Autodesk Inventor part; units mm, degrees
(part 2 of 3)
  spline S198 degree 2 poles (343.738, 65.1284) (343.9064, 65.1284) (344.2478, 65.1557) (344.571, 65.2012) (344.8623, 65.2604) (344.9852, 65.2968) knots 0 0 0 1 2 3 4 4 4
  line L272 (344.9852, 65.2968) -> (344.9852, 64.7415)
  spline S199 degree 2 poles (344.9852, 64.7415) (344.7076, 64.6641) (344.0111, 64.564) (343.6379, 64.564) knots 0 0 0 1 2 2 2
  spline S200 degree 2 poles (343.6379, 64.564) (343.1371, 64.564) (342.4134, 64.8371) (341.9536, 65.3515) (341.7306, 66.1025) (341.7306, 66.5759) knots 0 0 0 1 2 3 4 4 4
  spline S201 degree 2 poles (341.7306, 66.5759) (341.7306, 66.9902) (341.9673, 67.723) (342.4225, 68.2784) (343.0825, 68.6061) (343.5013, 68.6061) knots 0 0 0 1 2 3 4 4 4
  spline S202 degree 2 poles (343.5013, 68.6061) (343.911, 68.6061) (344.5437, 68.3512) (344.9716, 67.8778) (345.1946, 67.2087) (345.1946, 66.7899) knots 0 0 0 1 2 3 4 4 4
  spline S203 degree 2 poles (344.4891, 66.8855) (344.5027, 67.1449) (344.3753, 67.5774) (344.1158, 67.8915) (343.7289, 68.0644) (343.4694, 68.0644) knots 0 0 0 1 2 3 4 4 4
  spline S204 degree 2 poles (343.4694, 68.0644) (343.2509, 68.0644) (342.8822, 67.8915) (342.6182, 67.5819) (342.4543, 67.1449) (342.4361, 66.8855) knots 0 0 0 1 2 3 4 4 4
  line L273 (342.4361, 66.8855) -> (344.4891, 66.8855)
  spline S205 degree 2 poles (346.0777, 66.5031) (346.0777, 66.9993) (346.3508, 67.7731) (346.8515, 68.3057) (347.5525, 68.5834) (347.985, 68.5834) knots 0 0 0 1 2 3 4 4 4
  spline S206 degree 2 poles (347.985, 68.5834) (348.1716, 68.5834) (348.5358, 68.5378) (348.7087, 68.4878) knots 0 0 0 1 2 2 2
  line L274 (348.7087, 68.4878) -> (348.7087, 70.1265)
  line L275 (348.7087, 70.1265) -> (349.387, 70.1265)
  line L276 (349.387, 70.1265) -> (349.387, 64.6322)
  line L277 (349.387, 64.6322) -> (348.7816, 64.6322)
  line L278 (348.7816, 64.6322) -> (348.7588, 65.3742)
  spline S207 degree 2 poles (348.7588, 65.3742) (348.4766, 64.96) (347.8166, 64.564) (347.4296, 64.564) knots 0 0 0 1 2 2 2
  spline S208 degree 2 poles (347.4296, 64.564) (347.0973, 64.564) (346.5875, 64.8416) (346.2507, 65.3515) (346.0777, 66.0661) (346.0777, 66.5031) knots 0 0 0 1 2 3 4 4 4
  spline S209 degree 2 poles (346.7696, 66.5441) (346.7696, 65.8385) (347.1838, 65.1421) (347.5662, 65.1421) knots 0 0 0 1 2 2 2
  spline S210 degree 2 poles (347.5662, 65.1421) (347.8211, 65.1421) (348.3947, 65.6018) (348.7087, 66.0525) knots 0 0 0 1 2 2 2
  line L279 (348.7087, 66.0525) -> (348.7087, 67.8641)
  spline S211 degree 2 poles (348.7087, 67.8641) (348.5403, 67.9415) (348.1398, 68.0235) (347.9395, 68.0235) knots 0 0 0 1 2 2 2
  spline S212 degree 2 poles (347.9395, 68.0235) (347.3887, 68.0235) (346.7696, 67.3088) (346.7696, 66.5441) knots 0 0 0 1 2 2 2
  spline S213 degree 2 poles (358.3726, 66.6533) (358.3726, 66.1708) (358.104, 65.4015) (357.6124, 64.8689) (356.9023, 64.5867) (356.4608, 64.5867) knots 0 0 0 1 2 3 4 4 4
  spline S214 degree 2 poles (356.4608, 64.5867) (356.1148, 64.5867) (355.391, 64.7187) (355.036, 64.8644) knots 0 0 0 1 2 2 2
  line L280 (355.036, 64.8644) -> (355.036, 70.1265)
  line L281 (355.036, 70.1265) -> (355.7142, 70.1265)
  line L282 (355.7142, 70.1265) -> (355.7142, 68.6152)
  line L283 (355.7142, 68.6152) -> (355.6824, 67.8915)
  spline S215 degree 2 poles (355.6824, 67.8915) (355.9737, 68.2829) (356.6383, 68.6061) (357.0206, 68.6061) knots 0 0 0 1 2 2 2
  spline S216 degree 2 poles (357.0206, 68.6061) (357.3529, 68.6061) (357.8582, 68.3284) (358.1996, 67.8186) (358.3726, 67.0994) (358.3726, 66.6533) knots 0 0 0 1 2 3 4 4 4
  spline S217 degree 2 poles (357.6807, 66.6215) (357.6807, 66.931) (357.5896, 67.4408) (357.3985, 67.8095) (357.0935, 68.0144) (356.8841, 68.0144) knots 0 0 0 1 2 3 4 4 4
  spline S218 degree 2 poles (356.8841, 68.0144) (356.7566, 68.0144) (356.4926, 67.9324) (356.2058, 67.7412) (355.8918, 67.4272) (355.7142, 67.195) knots 0 0 0 1 2 3 4 4 4
  line L284 (355.7142, 67.195) -> (355.7142, 65.3014)
  spline S219 degree 2 poles (355.7142, 65.3014) (355.9145, 65.224) (356.3242, 65.133) (356.5108, 65.133) knots 0 0 0 1 2 2 2
  spline S220 degree 2 poles (356.5108, 65.133) (356.743, 65.133) (357.1663, 65.2786) (357.4895, 65.6246) (357.6807, 66.1981) (357.6807, 66.6215) knots 0 0 0 1 2 3 4 4 4
  line L285 (362.8881, 68.5333) -> (361.559, 65.0465)
  spline S221 degree 2 poles (361.559, 65.0465) (361.3496, 64.5139) (360.9126, 63.7446) (360.3891, 63.2484) (359.77, 63.0163) (359.3831, 63.0163) knots 0 0 0 1 2 3 4 4 4
  spline S222 degree 2 poles (359.3831, 63.0163) (359.283, 63.0163) (359.1191, 63.0254) (359.0235, 63.0345) knots 0 0 0 1 2 2 2
  line L286 (359.0235, 63.0345) -> (359.0235, 63.649)
  spline S223 degree 2 poles (359.0235, 63.649) (359.1055, 63.6354) (359.3103, 63.6172) (359.4241, 63.6172) knots 0 0 0 1 2 2 2
  spline S224 degree 2 poles (359.4241, 63.6172) (359.6107, 63.6172) (359.9339, 63.7264) (360.2207, 63.9677) (360.4847, 64.3591) (360.6076, 64.6322) knots 0 0 0 1 2 3 4 4 4
  line L287 (360.6076, 64.6322) -> (359.0508, 68.5333)
  line L288 (359.0508, 68.5333) -> (359.8201, 68.5333)
  line L289 (359.8201, 68.5333) -> (360.8079, 65.9523)
  line L290 (360.8079, 65.9523) -> (361.0082, 65.3469)
  line L291 (361.0082, 65.3469) -> (361.2312, 65.9705)
  line L292 (361.2312, 65.9705) -> (362.1416, 68.5333)
  line L293 (362.1416, 68.5333) -> (362.8881, 68.5333)
  line L294 (371.7508, 69.7122) -> (371.4094, 64.6322)
  line L295 (371.4094, 64.6322) -> (370.5127, 64.6322)
  line L296 (370.5127, 64.6322) -> (369.88, 66.4394)
  line L297 (369.88, 66.4394) -> (369.707, 67.0175)
  line L298 (369.707, 67.0175) -> (369.5249, 66.3939)
  line L299 (369.5249, 66.3939) -> (368.9377, 64.6322)
  line L300 (368.9377, 64.6322) -> (368.0728, 64.6322)
  line L301 (368.0728, 64.6322) -> (367.7223, 69.7122)
  line L302 (367.7223, 69.7122) -> (368.3733, 69.7122)
  line L303 (368.3733, 69.7122) -> (368.5736, 66.2527)
  line L304 (368.5736, 66.2527) -> (368.6327, 65.3059)
  line L305 (368.6327, 65.3059) -> (368.8785, 66.1116)
  line L306 (368.8785, 66.1116) -> (369.493, 67.9962)
  line L307 (369.493, 67.9962) -> (369.971, 67.9962)
  line L308 (369.971, 67.9962) -> (370.6811, 65.9751)
  line L309 (370.6811, 65.9751) -> (370.9178, 65.3059)
  line L310 (370.9178, 65.3059) -> (370.9315, 66.0024)
  line L311 (370.9315, 66.0024) -> (371.1318, 69.7122)
  line L312 (371.1318, 69.7122) -> (371.7508, 69.7122)
  line L313 (373.8811, 67.9734) -> (372.7249, 67.9734)
  line L314 (372.7249, 67.9734) -> (372.7249, 68.5333)
  line L315 (372.7249, 68.5333) -> (374.5639, 68.5333)
  line L316 (374.5639, 68.5333) -> (374.5639, 65.1967)
  line L317 (374.5639, 65.1967) -> (375.7247, 65.1967)
  line L318 (375.7247, 65.1967) -> (375.7247, 64.6322)
  line L319 (375.7247, 64.6322) -> (372.5975, 64.6322)
  line L320 (372.5975, 64.6322) -> (372.5975, 65.1967)
  line L321 (372.5975, 65.1967) -> (373.8811, 65.1967)
  line L322 (373.8811, 65.1967) -> (373.8811, 67.9734)
  spline S225 degree 2 poles (374.1179, 70.172) (374.2317, 70.172) (374.4228, 70.0901) (374.5685, 69.9444) (374.6504, 69.7532) (374.6504, 69.6394) knots 0 0 0 1 2 3 4 4 4
  spline S226 degree 2 poles (374.6504, 69.6394) (374.6504, 69.5302) (374.5685, 69.3344) (374.4228, 69.1888) (374.2317, 69.1068) (374.1179, 69.1068) knots 0 0 0 1 2 3 4 4 4
  spline S227 degree 2 poles (374.1179, 69.1068) (374.0041, 69.1068) (373.8129, 69.1888) (373.6672, 69.3344) (373.5853, 69.5302) (373.5853, 69.6394) knots 0 0 0 1 2 3 4 4 4
  spline S228 degree 2 poles (373.5853, 69.6394) (373.5853, 69.7532) (373.6672, 69.9444) (373.8129, 70.0901) (374.0041, 70.172) (374.1179, 70.172) knots 0 0 0 1 2 3 4 4 4
  line L323 (376.931, 68.5333) -> (377.5364, 68.5333)
  line L324 (377.5364, 68.5333) -> (377.5637, 67.9051)
  spline S229 degree 2 poles (377.5637, 67.9051) (377.7321, 68.1054) (378.0508, 68.374) (378.3603, 68.5378) (378.6789, 68.6061) (378.8519, 68.6061) knots 0 0 0 1 2 3 4 4 4
  spline S230 degree 2 poles (378.8519, 68.6061) (379.4528, 68.6061) (380.0718, 67.896) (380.0718, 67.1813) knots 0 0 0 1 2 2 2
  line L325 (380.0718, 67.1813) -> (380.0718, 64.6322)
  line L326 (380.0718, 64.6322) -> (379.3936, 64.6322)
  line L327 (379.3936, 64.6322) -> (379.3936, 67.1267)
  spline S231 degree 2 poles (379.3936, 67.1267) (379.3936, 67.5819) (379.0522, 68.0235) (378.7153, 68.0235) knots 0 0 0 1 2 2 2
  spline S232 degree 2 poles (378.7153, 68.0235) (378.5879, 68.0235) (378.3512, 67.9506) (378.0963, 67.7686) (377.7958, 67.4545) (377.6092, 67.2223) knots 0 0 0 1 2 3 4 4 4
  line L328 (377.6092, 67.2223) -> (377.6092, 64.6322)
  line L329 (377.6092, 64.6322) -> (376.931, 64.6322)
  line L330 (376.931, 64.6322) -> (376.931, 68.5333)
  spline S233 degree 2 poles (381.1097, 66.5031) (381.1097, 66.9993) (381.3828, 67.7731) (381.8835, 68.3057) (382.5845, 68.5834) (383.017, 68.5834) knots 0 0 0 1 2 3 4 4 4
  spline S234 degree 2 poles (383.017, 68.5834) (383.2036, 68.5834) (383.5677, 68.5378) (383.7407, 68.4878) knots 0 0 0 1 2 2 2
  line L331 (383.7407, 68.4878) -> (383.7407, 70.1265)
  line L332 (383.7407, 70.1265) -> (384.419, 70.1265)
  line L333 (384.419, 70.1265) -> (384.419, 64.6322)
  line L334 (384.419, 64.6322) -> (383.8136, 64.6322)
  line L335 (383.8136, 64.6322) -> (383.7908, 65.3742)
  spline S235 degree 2 poles (383.7908, 65.3742) (383.5086, 64.96) (382.8485, 64.564) (382.4616, 64.564) knots 0 0 0 1 2 2 2
  spline S236 degree 2 poles (382.4616, 64.564) (382.1293, 64.564) (381.6195, 64.8416) (381.2827, 65.3515) (381.1097, 66.0661) (381.1097, 66.5031) knots 0 0 0 1 2 3 4 4 4
  spline S237 degree 2 poles (381.8016, 66.5441) (381.8016, 65.8385) (382.2158, 65.1421) (382.5982, 65.1421) knots 0 0 0 1 2 2 2
  spline S238 degree 2 poles (382.5982, 65.1421) (382.8531, 65.1421) (383.4266, 65.6018) (383.7407, 66.0525) knots 0 0 0 1 2 2 2
  line L336 (383.7407, 66.0525) -> (383.7407, 67.8641)
  spline S239 degree 2 poles (383.7407, 67.8641) (383.5723, 67.9415) (383.1717, 68.0235) (382.9714, 68.0235) knots 0 0 0 1 2 2 2
  spline S240 degree 2 poles (382.9714, 68.0235) (382.4206, 68.0235) (381.8016, 67.3088) (381.8016, 66.5441) knots 0 0 0 1 2 2 2
  spline S241 degree 2 poles (389.2304, 67.2087) (389.2304, 66.5213) (388.9072, 65.529) (388.361, 64.8781) (387.6236, 64.564) (387.2184, 64.564) knots 0 0 0 1 2 3 4 4 4
  spline S242 degree 2 poles (387.2184, 64.564) (386.7268, 64.564) (385.9985, 64.919) (385.5205, 65.5882) (385.2884, 66.5486) (385.2884, 67.1495) knots 0 0 0 1 2 3 4 4 4
  spline S243 degree 2 poles (385.2884, 67.1495) (385.2884, 67.8277) (385.607, 68.8201) (386.1533, 69.471) (386.8861, 69.7851) (387.2958, 69.7851) knots 0 0 0 1 2 3 4 4 4
  spline S244 degree 2 poles (387.2958, 69.7851) (387.7829, 69.7851) (388.5112, 69.4255) (388.9937, 68.7609) (389.2304, 67.805) (389.2304, 67.2087) knots 0 0 0 1 2 3 4 4 4
  spline S245 degree 2 poles (388.5385, 67.1586) (388.5385, 67.6047) (388.3974, 68.3467) (388.0879, 68.8838) (387.6008, 69.1797) (387.2548, 69.1797) knots 0 0 0 1 2 3 4 4 4
  spline S246 degree 2 poles (387.2548, 69.1797) (386.9225, 69.1797) (386.44, 68.8656) (386.1305, 68.3239) (385.9803, 67.5956) (385.9803, 67.1859) knots 0 0 0 1 2 3 4 4 4
  spline S247 degree 2 poles (385.9803, 67.1859) (385.9803, 66.7353) (386.1214, 65.9933) (386.4309, 65.4607) (386.9134, 65.1648) (387.2548, 65.1648) knots 0 0 0 1 2 3 4 4 4
  spline S248 degree 2 poles (387.2548, 65.1648) (387.5871, 65.1648) (388.0742, 65.4789) (388.3883, 66.0206) (388.5385, 66.7444) (388.5385, 67.1586) knots 0 0 0 1 2 3 4 4 4
  spline S249 degree 2 poles (393.3181, 66.0115) (393.3181, 65.6473) (393.0222, 65.1056) (392.4942, 64.7415) (391.7522, 64.564) (391.3015, 64.564) knots 0 0 0 1 2 3 4 4 4
  spline S250 degree 2 poles (391.3015, 64.564) (391.1013, 64.564) (390.7007, 64.5958) (390.332, 64.6413) (390.0042, 64.7005) (389.8722, 64.7369) knots 0 0 0 1 2 3 4 4 4
  line L337 (389.8722, 64.7369) -> (389.8722, 65.4061)
  spline S251 degree 2 poles (389.8722, 65.4061) (390.1636, 65.2968) (390.8919, 65.1739) (391.3516, 65.1739) knots 0 0 0 1 2 2 2
  spline S252 degree 2 poles (391.3516, 65.1739) (391.6885, 65.1739) (392.1573, 65.2786) (392.4577, 65.4835) (392.5943, 65.7793) (392.5943, 65.9705) knots 0 0 0 1 2 3 4 4 4
  spline S253 degree 2 poles (392.5943, 65.9705) (392.5943, 66.1754) (392.3667, 66.4667) (391.9934, 66.6988) (391.5155, 66.89) (391.0148, 67.0903) (390.5368, 67.327) (390.1636, 67.6502) (389.936, 68.0872) (389.936, 68.3876) knots 0 0 0 1 2 3 4 5 6 7 8 8 8
  spline S254 degree 2 poles (389.936, 68.3876) (389.936, 68.6471) (390.1544, 69.1524) (390.6142, 69.5438) (391.3289, 69.7851) (391.8296, 69.7851) knots 0 0 0 1 2 3 4 4 4
  spline S255 degree 2 poles (391.8296, 69.7851) (391.957, 69.7851) (392.2575, 69.7623) (392.5624, 69.7213) (392.8629, 69.6667) (392.9903, 69.6349) knots 0 0 0 1 2 3 4 4 4
  line L338 (392.9903, 69.6349) -> (392.9903, 69.0112)
  spline S256 degree 2 poles (392.9903, 69.0112) (392.6899, 69.0977) (392.0936, 69.1842) (391.8114, 69.1842) knots 0 0 0 1 2 2 2
  spline S257 degree 2 poles (391.8114, 69.1842) (391.2196, 69.1842) (390.6597, 68.7882) (390.6597, 68.4559) knots 0 0 0 1 2 2 2
  spline S258 degree 2 poles (390.6597, 68.4559) (390.6597, 68.2511) (390.8873, 67.9552) (391.2606, 67.7185) (391.7385, 67.5319) (392.2393, 67.327) (392.7172, 67.0858) (393.0905, 66.758) (393.3181, 66.3119) (393.3181, 66.0115) knots 0 0 0 1 2 3 4 5 6 7 8 8 8
  line L339 (323.723, 56.0664) -> (322.9673, 56.0664)
  line L340 (322.9673, 56.0664) -> (322.6168, 57.1726)
  line L341 (322.6168, 57.1726) -> (320.4911, 57.1726)
  line L342 (320.4911, 57.1726) -> (320.136, 56.0664)
  line L343 (320.136, 56.0664) -> (319.4214, 56.0664)
  line L344 (319.4214, 56.0664) -> (321.1056, 61.1464)
  line L345 (321.1056, 61.1464) -> (322.057, 61.1464)
  line L346 (322.057, 61.1464) -> (323.723, 56.0664)
  line L347 (322.4166, 57.7916) -> (321.5562, 60.5137)
  line L348 (321.5562, 60.5137) -> (320.6868, 57.7916)
  line L349 (320.6868, 57.7916) -> (322.4166, 57.7916)
  spline S259 degree 2 poles (327.4692, 57.1316) (327.4692, 56.9268) (327.3281, 56.599) (327.0869, 56.3487) (326.7682, 56.1711) (326.4086, 56.0528) (326.0263, 55.9982) (325.8442, 55.9982) knots 0 0 0 1 2 3 4 5 6 6 6
  spline S260 degree 2 poles (325.8442, 55.9982) (325.4482, 55.9982) (324.7836, 56.071) (324.4649, 56.1484) knots 0 0 0 1 2 2 2
  line L350 (324.4649, 56.1484) -> (324.4649, 56.772)
  spline S261 degree 2 poles (324.4649, 56.772) (324.8063, 56.6718) (325.4846, 56.5717) (325.8169, 56.5717) knots 0 0 0 1 2 2 2
  spline S262 degree 2 poles (325.8169, 56.5717) (326.3039, 56.5717) (326.7682, 56.8357) (326.7682, 57.077) knots 0 0 0 1 2 2 2
  spline S263 degree 2 poles (326.7682, 57.077) (326.7682, 57.1817) (326.6954, 57.3501) (326.4997, 57.5003) (326.0946, 57.6642) (325.7395, 57.7689) knots 0 0 0 1 2 3 4 4 4
  spline S264 degree 2 poles (325.7395, 57.7689) (325.4755, 57.8463) (325.0294, 58.0465) (324.7016, 58.3197) (324.515, 58.6838) (324.515, 58.9342) knots 0 0 0 1 2 3 4 4 4
  spline S265 degree 2 poles (324.515, 58.9342) (324.515, 59.098) (324.6652, 59.485) (325.0339, 59.8173) (325.653, 60.0403) (326.1219, 60.0403) knots 0 0 0 1 2 3 4 4 4
  spline S266 degree 2 poles (326.1219, 60.0403) (326.3495, 60.0403) (326.9094, 59.9902) (327.2143, 59.9265) knots 0 0 0 1 2 2 2
  line L351 (327.2143, 59.9265) -> (327.2143, 59.3256)
  spline S267 degree 2 poles (327.2143, 59.3256) (326.8957, 59.403) (326.3222, 59.4759) (326.1128, 59.4759) knots 0 0 0 1 2 2 2
  spline S268 degree 2 poles (326.1128, 59.4759) (325.8624, 59.4759) (325.5165, 59.3985) (325.3025, 59.2619) (325.2069, 59.0798) (325.2069, 58.9751) knots 0 0 0 1 2 3 4 4 4
  spline S269 degree 2 poles (325.2069, 58.9751) (325.2069, 58.8704) (325.2889, 58.6975) (325.5119, 58.5382) (325.9079, 58.3788) (326.2266, 58.2878) knots 0 0 0 1 2 3 4 4 4
  spline S270 degree 2 poles (326.2266, 58.2878) (326.5725, 58.1877) (327.0459, 57.9646) (327.3418, 57.6915) (327.4692, 57.3501) (327.4692, 57.1316) knots 0 0 0 1 2 3 4 4 4
  spline S271 degree 2 poles (331.8482, 57.1316) (331.8482, 56.9268) (331.7071, 56.599) (331.4659, 56.3487) (331.1472, 56.1711) (330.7876, 56.0528) (330.4053, 55.9982) (330.2232, 55.9982) knots 0 0 0 1 2 3 4 5 6 6 6
  spline S272 degree 2 poles (330.2232, 55.9982) (329.8272, 55.9982) (329.1626, 56.071) (328.8439, 56.1484) knots 0 0 0 1 2 2 2
  line L352 (328.8439, 56.1484) -> (328.8439, 56.772)
  spline S273 degree 2 poles (328.8439, 56.772) (329.1853, 56.6718) (329.8636, 56.5717) (330.1959, 56.5717) knots 0 0 0 1 2 2 2
  spline S274 degree 2 poles (330.1959, 56.5717) (330.6829, 56.5717) (331.1472, 56.8357) (331.1472, 57.077) knots 0 0 0 1 2 2 2
  spline S275 degree 2 poles (331.1472, 57.077) (331.1472, 57.1817) (331.0744, 57.3501) (330.8787, 57.5003) (330.4735, 57.6642) (330.1185, 57.7689) knots 0 0 0 1 2 3 4 4 4
  spline S276 degree 2 poles (330.1185, 57.7689) (329.8545, 57.8463) (329.4084, 58.0465) (329.0806, 58.3197) (328.894, 58.6838) (328.894, 58.9342) knots 0 0 0 1 2 3 4 4 4
  spline S277 degree 2 poles (328.894, 58.9342) (328.894, 59.098) (329.0442, 59.485) (329.4129, 59.8173) (330.032, 60.0403) (330.5009, 60.0403) knots 0 0 0 1 2 3 4 4 4
  spline S278 degree 2 poles (330.5009, 60.0403) (330.7285, 60.0403) (331.2884, 59.9902) (331.5933, 59.9265) knots 0 0 0 1 2 2 2
  line L353 (331.5933, 59.9265) -> (331.5933, 59.3256)
  spline S279 degree 2 poles (331.5933, 59.3256) (331.2747, 59.403) (330.7011, 59.4759) (330.4918, 59.4759) knots 0 0 0 1 2 2 2
  spline S280 degree 2 poles (330.4918, 59.4759) (330.2414, 59.4759) (329.8954, 59.3985) (329.6815, 59.2619) (329.5859, 59.0798) (329.5859, 58.9751) knots 0 0 0 1 2 3 4 4 4
  spline S281 degree 2 poles (329.5859, 58.9751) (329.5859, 58.8704) (329.6679, 58.6975) (329.8909, 58.5382) (330.2869, 58.3788) (330.6056, 58.2878) knots 0 0 0 1 2 3 4 4 4
  spline S282 degree 2 poles (330.6056, 58.2878) (330.9515, 58.1877) (331.4249, 57.9646) (331.7208, 57.6915) (331.8482, 57.3501) (331.8482, 57.1316) knots 0 0 0 1 2 3 4 4 4
  spline S283 degree 2 poles (336.4366, 58.2241) (336.4366, 58.083) (336.4275, 57.8872) (336.423, 57.8007) knots 0 0 0 1 2 2 2
  line L354 (336.423, 57.8007) -> (333.6781, 57.8007)
  spline S284 degree 2 poles (333.6781, 57.8007) (333.6781, 57.2044) (334.3473, 56.5626) (334.98, 56.5626) knots 0 0 0 1 2 2 2
  spline S285 degree 2 poles (334.98, 56.5626) (335.1484, 56.5626) (335.4898, 56.5899) (335.813, 56.6354) (336.1043, 56.6946) (336.2272, 56.731) knots 0 0 0 1 2 3 4 4 4
  line L355 (336.2272, 56.731) -> (336.2272, 56.1757)
  spline S286 degree 2 poles (336.2272, 56.1757) (335.9496, 56.0983) (335.2531, 55.9982) (334.8799, 55.9982) knots 0 0 0 1 2 2 2
  spline S287 degree 2 poles (334.8799, 55.9982) (334.3791, 55.9982) (333.6554, 56.2713) (333.1956, 56.7856) (332.9726, 57.5367) (332.9726, 58.0101) knots 0 0 0 1 2 3 4 4 4
  spline S288 degree 2 poles (332.9726, 58.0101) (332.9726, 58.4244) (333.2093, 59.1572) (333.6645, 59.7126) (334.3245, 60.0403) (334.7433, 60.0403) knots 0 0 0 1 2 3 4 4 4
  spline S289 degree 2 poles (334.7433, 60.0403) (335.153, 60.0403) (335.7857, 59.7854) (336.2136, 59.312) (336.4366, 58.6428) (336.4366, 58.2241) knots 0 0 0 1 2 3 4 4 4
  spline S290 degree 2 poles (335.7311, 58.3197) (335.7447, 58.5791) (335.6173, 59.0116) (335.3578, 59.3256) (334.9709, 59.4986) (334.7114, 59.4986) knots 0 0 0 1 2 3 4 4 4
  spline S291 degree 2 poles (334.7114, 59.4986) (334.4929, 59.4986) (334.1242, 59.3256) (333.8602, 59.0161) (333.6963, 58.5791) (333.6781, 58.3197) knots 0 0 0 1 2 3 4 4 4
  line L356 (333.6781, 58.3197) -> (335.7311, 58.3197)
  line L357 (340.3058, 56.0664) -> (340.3058, 58.8704)
  spline S292 degree 2 poles (340.3058, 58.8704) (340.3058, 59.0525) (340.2785, 59.2847) (340.2239, 59.4212) (340.1419, 59.4759) (340.0782, 59.4759) knots 0 0 0 1 2 3 4 4 4
  spline S293 degree 2 poles (340.0782, 59.4759) (340.0054, 59.4759) (339.8825, 59.3848) (339.7414, 59.1709) (339.5729, 58.8249) (339.4546, 58.5746) knots 0 0 0 1 2 3 4 4 4
  line L358 (339.4546, 58.5746) -> (339.4546, 56.0664)
  line L359 (339.4546, 56.0664) -> (338.7763, 56.0664)
  line L360 (338.7763, 56.0664) -> (338.7763, 58.7976)
  spline S294 degree 2 poles (338.7763, 58.7976) (338.7763, 59.0116) (338.749, 59.2756) (338.6944, 59.4212) (338.6079, 59.4759) (338.5442, 59.4759) knots 0 0 0 1 2 3 4 4 4
  spline S295 degree 2 poles (338.5442, 59.4759) (338.4805, 59.4759) (338.3621, 59.3985) (338.221, 59.1982) (338.0435, 58.8477) (337.9251, 58.5746) knots 0 0 0 1 2 3 4 4 4
  line L361 (337.9251, 58.5746) -> (337.9251, 56.0664)
  line L362 (337.9251, 56.0664) -> (337.2469, 56.0664)
  line L363 (337.2469, 56.0664) -> (337.2469, 59.9675)
  line L364 (337.2469, 59.9675) -> (337.8113, 59.9675)
  line L365 (337.8113, 59.9675) -> (337.8432, 59.2255)
  spline S296 degree 2 poles (337.8432, 59.2255) (337.9479, 59.4485) (338.1391, 59.7581) (338.3394, 59.9493) (338.5715, 60.0403) (338.7081, 60.0403) knots 0 0 0 1 2 3 4 4 4
  spline S297 degree 2 poles (338.7081, 60.0403) (339.0267, 60.0403) (339.3544, 59.6261) (339.3544, 59.1936) knots 0 0 0 1 2 2 2
  spline S298 degree 2 poles (339.3544, 59.1936) (339.4455, 59.3985) (339.6276, 59.7126) (339.8324, 59.9265) (340.0828, 60.0403) (340.2466, 60.0403) knots 0 0 0 1 2 3 4 4 4
  spline S299 degree 2 poles (340.2466, 60.0403) (340.9841, 60.0403) (340.9841, 58.9069) knots 0 0 0 1 1 1
  line L366 (340.9841, 58.9069) -> (340.9841, 56.0664)
  line L367 (340.9841, 56.0664) -> (340.3058, 56.0664)
  spline S300 degree 2 poles (345.2356, 58.0875) (345.2356, 57.605) (344.967, 56.8357) (344.4754, 56.3031) (343.7653, 56.0209) (343.3238, 56.0209) knots 0 0 0 1 2 3 4 4 4
  spline S301 degree 2 poles (343.3238, 56.0209) (342.9778, 56.0209) (342.2541, 56.1529) (341.899, 56.2986) knots 0 0 0 1 2 2 2
  line L368 (341.899, 56.2986) -> (341.899, 61.5607)
  line L369 (341.899, 61.5607) -> (342.5772, 61.5607)
  line L370 (342.5772, 61.5607) -> (342.5772, 60.0494)
  line L371 (342.5772, 60.0494) -> (342.5454, 59.3256)
  spline S302 degree 2 poles (342.5454, 59.3256) (342.8367, 59.7171) (343.5013, 60.0403) (343.8837, 60.0403) knots 0 0 0 1 2 2 2
  spline S303 degree 2 poles (343.8837, 60.0403) (344.216, 60.0403) (344.7212, 59.7626) (345.0626, 59.2528) (345.2356, 58.5336) (345.2356, 58.0875) knots 0 0 0 1 2 3 4 4 4
  spline S304 degree 2 poles (344.5437, 58.0556) (344.5437, 58.3652) (344.4527, 58.875) (344.2615, 59.2437) (343.9565, 59.4485) (343.7471, 59.4485) knots 0 0 0 1 2 3 4 4 4
  spline S305 degree 2 poles (343.7471, 59.4485) (343.6196, 59.4485) (343.3556, 59.3666) (343.0689, 59.1754) (342.7548, 58.8613) (342.5772, 58.6292) knots 0 0 0 1 2 3 4 4 4
  line L372 (342.5772, 58.6292) -> (342.5772, 56.7356)
  spline S306 degree 2 poles (342.5772, 56.7356) (342.7775, 56.6582) (343.1872, 56.5672) (343.3738, 56.5672) knots 0 0 0 1 2 2 2
  spline S307 degree 2 poles (343.3738, 56.5672) (343.606, 56.5672) (344.0293, 56.7128) (344.3525, 57.0588) (344.5437, 57.6323) (344.5437, 58.0556) knots 0 0 0 1 2 3 4 4 4
  line L373 (347.6072, 61.0053) -> (346.451, 61.0053)
  line L374 (346.451, 61.0053) -> (346.451, 61.5607)
  line L375 (346.451, 61.5607) -> (348.29, 61.5607)
  line L376 (348.29, 61.5607) -> (348.29, 56.6309)
  line L377 (348.29, 56.6309) -> (349.4507, 56.6309)
  line L378 (349.4507, 56.6309) -> (349.4507, 56.0664)
  line L379 (349.4507, 56.0664) -> (346.3235, 56.0664)
  line L380 (346.3235, 56.0664) -> (346.3235, 56.6309)
  line L381 (346.3235, 56.6309) -> (347.6072, 56.6309)
  line L382 (347.6072, 56.6309) -> (347.6072, 61.0053)
  spline S308 degree 2 poles (353.9526, 58.2241) (353.9526, 58.083) (353.9435, 57.8872) (353.939, 57.8007) knots 0 0 0 1 2 2 2
  line L383 (353.939, 57.8007) -> (351.1941, 57.8007)
  spline S309 degree 2 poles (351.1941, 57.8007) (351.1941, 57.2044) (351.8633, 56.5626) (352.496, 56.5626) knots 0 0 0 1 2 2 2
  spline S310 degree 2 poles (352.496, 56.5626) (352.6644, 56.5626) (353.0058, 56.5899) (353.329, 56.6354) (353.6203, 56.6946) (353.7432, 56.731) knots 0 0 0 1 2 3 4 4 4
  line L384 (353.7432, 56.731) -> (353.7432, 56.1757)
  spline S311 degree 2 poles (353.7432, 56.1757) (353.4656, 56.0983) (352.7691, 55.9982) (352.3958, 55.9982) knots 0 0 0 1 2 2 2
  spline S312 degree 2 poles (352.3958, 55.9982) (351.8951, 55.9982) (351.1714, 56.2713) (350.7116, 56.7856) (350.4886, 57.5367) (350.4886, 58.0101) knots 0 0 0 1 2 3 4 4 4
  spline S313 degree 2 poles (350.4886, 58.0101) (350.4886, 58.4244) (350.7253, 59.1572) (351.1805, 59.7126) (351.8405, 60.0403) (352.2593, 60.0403) knots 0 0 0 1 2 3 4 4 4
  spline S314 degree 2 poles (352.2593, 60.0403) (352.669, 60.0403) (353.3017, 59.7854) (353.7296, 59.312) (353.9526, 58.6428) (353.9526, 58.2241) knots 0 0 0 1 2 3 4 4 4
  spline S315 degree 2 poles (353.2471, 58.3197) (353.2607, 58.5791) (353.1333, 59.0116) (352.8738, 59.3256) (352.4869, 59.4986) (352.2274, 59.4986) knots 0 0 0 1 2 3 4 4 4
  spline S316 degree 2 poles (352.2274, 59.4986) (352.0089, 59.4986) (351.6402, 59.3256) (351.3762, 59.0161) (351.2123, 58.5791) (351.1941, 58.3197) knots 0 0 0 1 2 3 4 4 4
  line L385 (351.1941, 58.3197) -> (353.2471, 58.3197)
  spline S317 degree 2 poles (354.8357, 57.9373) (354.8357, 58.4335) (355.1088, 59.2073) (355.6095, 59.7399) (356.3105, 60.0175) (356.743, 60.0175) knots 0 0 0 1 2 3 4 4 4
  spline S318 degree 2 poles (356.743, 60.0175) (356.9296, 60.0175) (357.2938, 59.972) (357.4667, 59.922) knots 0 0 0 1 2 2 2
  line L386 (357.4667, 59.922) -> (357.4667, 61.5607)
  line L387 (357.4667, 61.5607) -> (358.145, 61.5607)
  line L388 (358.145, 61.5607) -> (358.145, 56.0664)
  line L389 (358.145, 56.0664) -> (357.5396, 56.0664)
  line L390 (357.5396, 56.0664) -> (357.5168, 56.8084)
  spline S319 degree 2 poles (357.5168, 56.8084) (357.2346, 56.3942) (356.5746, 55.9982) (356.1876, 55.9982) knots 0 0 0 1 2 2 2
  spline S320 degree 2 poles (356.1876, 55.9982) (355.8553, 55.9982) (355.3455, 56.2758) (355.0087, 56.7856) (354.8357, 57.5003) (354.8357, 57.9373) knots 0 0 0 1 2 3 4 4 4
  spline S321 degree 2 poles (355.5276, 57.9783) (355.5276, 57.2727) (355.9418, 56.5763) (356.3242, 56.5763) knots 0 0 0 1 2 2 2
  spline S322 degree 2 poles (356.3242, 56.5763) (356.5791, 56.5763) (357.1527, 57.036) (357.4667, 57.4866) knots 0 0 0 1 2 2 2
  line L391 (357.4667, 57.4866) -> (357.4667, 59.2983)
  spline S323 degree 2 poles (357.4667, 59.2983) (357.2983, 59.3757) (356.8977, 59.4577) (356.6975, 59.4577) knots 0 0 0 1 2 2 2
  spline S324 degree 2 poles (356.6975, 59.4577) (356.1467, 59.4577) (355.5276, 58.743) (355.5276, 57.9783) knots 0 0 0 1 2 2 2
  line L392 (367.258, 56.0664) -> (366.4751, 56.0664)
  line L393 (366.4751, 56.0664) -> (365.7149, 57.6915)
  spline S325 degree 2 poles (365.7149, 57.6915) (365.633, 57.8781) (365.4509, 58.1239) (365.2461, 58.265) (365.0003, 58.3288) (364.85, 58.3288) knots 0 0 0 1 2 3 4 4 4
  line L394 (364.85, 58.3288) -> (364.5223, 58.3288)
  line L395 (364.5223, 58.3288) -> (364.5223, 56.0664)
  line L396 (364.5223, 56.0664) -> (363.8304, 56.0664)
  line L397 (363.8304, 56.0664) -> (363.8304, 61.1464)
  line L398 (363.8304, 61.1464) -> (365.1914, 61.1464)
  spline S326 degree 2 poles (365.1914, 61.1464) (365.633, 61.1464) (366.2703, 60.9507) (366.6799, 60.6002) (366.8711, 60.1086) (366.8711, 59.8082) knots 0 0 0 1 2 3 4 4 4
  spline S327 degree 2 poles (366.8711, 59.8082) (366.8711, 59.5715) (366.73, 59.1481) (366.4569, 58.8022) (366.0472, 58.5518) (365.7832, 58.4881) knots 0 0 0 1 2 3 4 4 4
  spline S328 degree 2 poles (365.7832, 58.4881) (365.9971, 58.4153) (366.2976, 58.0465) (366.4523, 57.737) knots 0 0 0 1 2 2 2
  line L399 (366.4523, 57.737) -> (367.258, 56.0664)
  spline S329 degree 2 poles (366.1473, 59.749) (366.1473, 60.1587) (365.6375, 60.5638) (365.1732, 60.5638) knots 0 0 0 1 2 2 2
  line L400 (365.1732, 60.5638) -> (364.5223, 60.5638)
  line L401 (364.5223, 60.5638) -> (364.5223, 58.8841)
  line L402 (364.5223, 58.8841) -> (365.0822, 58.8841)
  spline S330 degree 2 poles (365.0822, 58.8841) (365.328, 58.8841) (365.7195, 58.9979) (365.9971, 59.2164) (366.1473, 59.5396) (366.1473, 59.749) knots 0 0 0 1 2 3 4 4 4
  line L403 (369.5022, 59.4076) -> (368.346, 59.4076)
  line L404 (368.346, 59.4076) -> (368.346, 59.9675)
  line L405 (368.346, 59.9675) -> (370.1849, 59.9675)
  line L406 (370.1849, 59.9675) -> (370.1849, 56.6309)
  line L407 (370.1849, 56.6309) -> (371.3457, 56.6309)
  line L408 (371.3457, 56.6309) -> (371.3457, 56.0664)
  line L409 (371.3457, 56.0664) -> (368.2185, 56.0664)
  line L410 (368.2185, 56.0664) -> (368.2185, 56.6309)
  line L411 (368.2185, 56.6309) -> (369.5022, 56.6309)
  line L412 (369.5022, 56.6309) -> (369.5022, 59.4076)
  spline S331 degree 2 poles (369.7389, 61.6062) (369.8527, 61.6062) (370.0438, 61.5242) (370.1895, 61.3786) (370.2714, 61.1874) (370.2714, 61.0736) knots 0 0 0 1 2 3 4 4 4
  spline S332 degree 2 poles (370.2714, 61.0736) (370.2714, 60.9644) (370.1895, 60.7686) (370.0438, 60.623) (369.8527, 60.541) (369.7389, 60.541) knots 0 0 0 1 2 3 4 4 4
  spline S333 degree 2 poles (369.7389, 60.541) (369.6251, 60.541) (369.4339, 60.623) (369.2882, 60.7686) (369.2063, 60.9644) (369.2063, 61.0736) knots 0 0 0 1 2 3 4 4 4
  spline S334 degree 2 poles (369.2063, 61.0736) (369.2063, 61.1874) (369.2882, 61.3786) (369.4339, 61.5242) (369.6251, 61.6062) (369.7389, 61.6062) knots 0 0 0 1 2 3 4 4 4
  spline S335 degree 2 poles (375.5836, 56.2121) (375.3196, 56.112) (374.7642, 56.0118) (374.4684, 56.0118) knots 0 0 0 1 2 2 2
  spline S336 degree 2 poles (374.4684, 56.0118) (373.5443, 56.0118) (372.5429, 57.0132) (372.5429, 57.9783) knots 0 0 0 1 2 2 2
  spline S337 degree 2 poles (372.5429, 57.9783) (372.5429, 58.4426) (372.8296, 59.1936) (373.3531, 59.7308) (374.0769, 60.0221) (374.5093, 60.0221) knots 0 0 0 1 2 3 4 4 4
  spline S338 degree 2 poles (374.5093, 60.0221) (374.8143, 60.0221) (375.3423, 59.9356) (375.5836, 59.84) knots 0 0 0 1 2 2 2
  line L413 (375.5836, 59.84) -> (375.5836, 59.1936)
  spline S339 degree 2 poles (375.5836, 59.1936) (375.3287, 59.3256) (374.8052, 59.4485) (374.523, 59.4485) knots 0 0 0 1 2 2 2
  spline S340 degree 2 poles (374.523, 59.4485) (374.2635, 59.4485) (373.7992, 59.2483) (373.4487, 58.875) (373.2484, 58.3379) (373.2484, 58.001) knots 0 0 0 1 2 3 4 4 4
  spline S341 degree 2 poles (373.2484, 58.001) (373.2484, 57.2955) (373.9358, 56.5899) (374.5503, 56.5899) knots 0 0 0 1 2 2 2
  spline S342 degree 2 poles (374.5503, 56.5899) (374.8234, 56.5899) (375.3423, 56.7174) (375.5836, 56.8403) knots 0 0 0 1 2 2 2
  line L414 (375.5836, 56.8403) -> (375.5836, 56.2121)
  line L415 (380.0718, 56.0664) -> (379.3936, 56.0664)
  line L416 (379.3936, 56.0664) -> (379.3936, 58.5609)
  spline S343 degree 2 poles (379.3936, 58.5609) (379.3936, 59.0116) (379.0567, 59.4577) (378.7427, 59.4577) knots 0 0 0 1 2 2 2
  spline S344 degree 2 poles (378.7427, 59.4577) (378.6061, 59.4577) (378.3694, 59.3848) (378.1099, 59.2027) (377.8095, 58.8887) (377.6092, 58.6565) knots 0 0 0 1 2 3 4 4 4
  line L417 (377.6092, 58.6565) -> (377.6092, 56.0664)
  line L418 (377.6092, 56.0664) -> (376.931, 56.0664)
  line L419 (376.931, 56.0664) -> (376.931, 61.5607)
  line L420 (376.931, 61.5607) -> (377.6092, 61.5607)
  line L421 (377.6092, 61.5607) -> (377.6092, 59.972)
  line L422 (377.6092, 59.972) -> (377.5865, 59.3575)
  spline S345 degree 2 poles (377.5865, 59.3575) (377.7458, 59.5487) (378.0508, 59.8082) (378.3603, 59.972) (378.6789, 60.0403) (378.8519, 60.0403) knots 0 0 0 1 2 3 4 4 4
  spline S346 degree 2 poles (378.8519, 60.0403) (379.4346, 60.0403) (380.0718, 59.3302) (380.0718, 58.6155) knots 0 0 0 1 2 2 2
  line L423 (380.0718, 58.6155) -> (380.0718, 56.0664)
  line L424 (382.6391, 61.0053) -> (381.4829, 61.0053)
  line L425 (381.4829, 61.0053) -> (381.4829, 61.5607)
  line L426 (381.4829, 61.5607) -> (383.3219, 61.5607)
  line L427 (383.3219, 61.5607) -> (383.3219, 56.6309)
  line L428 (383.3219, 56.6309) -> (384.4827, 56.6309)
  line L429 (384.4827, 56.6309) -> (384.4827, 56.0664)
  line L430 (384.4827, 56.0664) -> (381.3555, 56.0664)
  line L431 (381.3555, 56.0664) -> (381.3555, 56.6309)
  line L432 (381.3555, 56.6309) -> (382.6391, 56.6309)
  line L433 (382.6391, 56.6309) -> (382.6391, 61.0053)
  line L434 (388.1971, 56.0664) -> (388.1834, 56.5899)
  spline S347 degree 2 poles (388.1834, 56.5899) (387.8648, 56.2758) (387.2048, 55.9982) (386.8452, 55.9982) knots 0 0 0 1 2 2 2
  spline S348 degree 2 poles (386.8452, 55.9982) (386.5083, 55.9982) (386.0349, 56.1711) (385.7299, 56.467) (385.5843, 56.8721) (385.5843, 57.1088) knots 0 0 0 1 2 3 4 4 4
  spline S349 degree 2 poles (385.5843, 57.1088) (385.5843, 57.696) (386.4582, 58.3606) (387.314, 58.3606) knots 0 0 0 1 2 2 2
  line L435 (387.314, 58.3606) -> (388.1243, 58.3606)
  line L436 (388.1243, 58.3606) -> (388.1243, 58.702)
  spline S350 degree 2 poles (388.1243, 58.702) (388.1243, 59.048) (387.6827, 59.4668) (387.2275, 59.4668) knots 0 0 0 1 2 2 2
  spline S351 degree 2 poles (387.2275, 59.4668) (386.8952, 59.4668) (386.2534, 59.3211) (385.912, 59.1845) knots 0 0 0 1 2 2 2
  line L437 (385.912, 59.1845) -> (385.912, 59.7945)
  spline S352 degree 2 poles (385.912, 59.7945) (386.0395, 59.84) (386.3536, 59.9311) (386.7041, 59.9993) (387.0864, 60.0403) (387.2776, 60.0403) knots 0 0 0 1 2 3 4 4 4
  spline S353 degree 2 poles (387.2776, 60.0403) (387.6327, 60.0403) (388.2017, 59.8855) (388.5931, 59.5669) (388.8025, 59.0844) (388.8025, 58.7566) knots 0 0 0 1 2 3 4 4 4
  line L438 (388.8025, 58.7566) -> (388.8025, 56.0664)
  line L439 (388.8025, 56.0664) -> (388.1971, 56.0664)
  line L440 (388.1243, 57.8417) -> (387.2639, 57.8417)
  spline S354 degree 2 poles (387.2639, 57.8417) (387.009, 57.8417) (386.6449, 57.7416) (386.4127, 57.5549) (386.2989, 57.2955) (386.2989, 57.1316) knots 0 0 0 1 2 3 4 4 4
  spline S355 degree 2 poles (386.2989, 57.1316) (386.2989, 57.0178) (386.3672, 56.813) (386.5265, 56.6536) (386.7723, 56.5626) (386.9544, 56.5626) knots 0 0 0 1 2 3 4 4 4
  spline S356 degree 2 poles (386.9544, 56.5626) (387.1866, 56.5626) (387.7874, 56.8448) (388.1243, 57.1498) knots 0 0 0 1 2 2 2
  line L441 (388.1243, 57.1498) -> (388.1243, 57.8417)
  line L442 (390.068, 59.9675) -> (390.6734, 59.9675)
  line L443 (390.6734, 59.9675) -> (390.7007, 59.3393)
  spline S357 degree 2 poles (390.7007, 59.3393) (390.8691, 59.5396) (391.1877, 59.8082) (391.4973, 59.972) (391.8159, 60.0403) (391.9889, 60.0403) knots 0 0 0 1 2 3 4 4 4
  spline S358 degree 2 poles (391.9889, 60.0403) (392.5898, 60.0403) (393.2088, 59.3302) (393.2088, 58.6155) knots 0 0 0 1 2 2 2
  line L444 (393.2088, 58.6155) -> (393.2088, 56.0664)
  line L445 (393.2088, 56.0664) -> (392.5306, 56.0664)
  line L446 (392.5306, 56.0664) -> (392.5306, 58.5609)
  spline S359 degree 2 poles (392.5306, 58.5609) (392.5306, 59.0161) (392.1892, 59.4577) (391.8523, 59.4577) knots 0 0 0 1 2 2 2
  spline S360 degree 2 poles (391.8523, 59.4577) (391.7249, 59.4577) (391.4882, 59.3848) (391.2333, 59.2027) (390.9328, 58.8887) (390.7462, 58.6565) knots 0 0 0 1 2 3 4 4 4
  line L447 (390.7462, 58.6565) -> (390.7462, 56.0664)
  line L448 (390.7462, 56.0664) -> (390.068, 56.0664)
  line L449 (390.068, 56.0664) -> (390.068, 59.9675)
  spline S361 degree 2 poles (394.2467, 57.9373) (394.2467, 58.4335) (394.5198, 59.2073) (395.0205, 59.7399) (395.7215, 60.0175) (396.1539, 60.0175) knots 0 0 0 1 2 3 4 4 4
  spline S362 degree 2 poles (396.1539, 60.0175) (396.3406, 60.0175) (396.7047, 59.972) (396.8777, 59.922) knots 0 0 0 1 2 2 2
  line L450 (396.8777, 59.922) -> (396.8777, 61.5607)
  line L451 (396.8777, 61.5607) -> (397.556, 61.5607)
  line L452 (397.556, 61.5607) -> (397.556, 56.0664)
  line L453 (397.556, 56.0664) -> (396.9505, 56.0664)
  line L454 (396.9505, 56.0664) -> (396.9278, 56.8084)
  spline S363 degree 2 poles (396.9278, 56.8084) (396.6456, 56.3942) (395.9855, 55.9982) (395.5986, 55.9982) knots 0 0 0 1 2 2 2
  spline S364 degree 2 poles (395.5986, 55.9982) (395.2663, 55.9982) (394.7565, 56.2758) (394.4196, 56.7856) (394.2467, 57.5003) (394.2467, 57.9373) knots 0 0 0 1 2 3 4 4 4
  spline S365 degree 2 poles (394.9386, 57.9783) (394.9386, 57.2727) (395.3528, 56.5763) (395.7352, 56.5763) knots 0 0 0 1 2 2 2
  spline S366 degree 2 poles (395.7352, 56.5763) (395.9901, 56.5763) (396.5636, 57.036) (396.8777, 57.4866) knots 0 0 0 1 2 2 2
  line L455 (396.8777, 57.4866) -> (396.8777, 59.2983)
  spline S367 degree 2 poles (396.8777, 59.2983) (396.7093, 59.3757) (396.3087, 59.4577) (396.1084, 59.4577) knots 0 0 0 1 2 2 2
  spline S368 degree 2 poles (396.1084, 59.4577) (395.5576, 59.4577) (394.9386, 58.743) (394.9386, 57.9783) knots 0 0 0 1 2 2 2
  spline S369 degree 2 poles (399.1264, 55.2698) (399.3267, 55.2607) (399.6954, 55.3472) (399.9822, 55.5156) (400.1506, 55.7615) (400.1506, 55.9208) knots 0 0 0 1 2 3 4 4 4
  spline S370 degree 2 poles (400.1506, 55.9208) (400.1506, 56.0846) (400.0413, 56.2849) (399.9002, 56.4579) (399.7864, 56.6536) (399.7864, 56.8175) knots 0 0 0 1 2 3 4 4 4
  spline S371 degree 2 poles (399.7864, 56.8175) (399.7864, 56.8994) (399.8501, 57.077) (399.9776, 57.2226) (400.1733, 57.3182) (400.3099, 57.3182) knots 0 0 0 1 2 3 4 4 4
  spline S372 degree 2 poles (400.3099, 57.3182) (400.4465, 57.3182) (400.6968, 57.2044) (400.888, 56.9723) (401.0018, 56.6218) (401.0018, 56.3851) knots 0 0 0 1 2 3 4 4 4
  spline S373 degree 2 poles (401.0018, 56.3851) (401.0018, 56.0619) (400.7651, 55.4701) (400.2962, 55.0104) (399.5907, 54.7373) (399.1264, 54.7373) knots 0 0 0 1 2 3 4 4 4
  line L456 (399.1264, 54.7373) -> (399.1264, 55.2698)
  line L457 (411.1618, 61.1464) -> (410.8204, 56.0664)
  line L458 (410.8204, 56.0664) -> (409.9237, 56.0664)
  line L459 (409.9237, 56.0664) -> (409.2909, 57.8736)
  line L460 (409.2909, 57.8736) -> (409.118, 58.4517)
  line L461 (409.118, 58.4517) -> (408.9359, 57.828)
  line L462 (408.9359, 57.828) -> (408.3487, 56.0664)
  line L463 (408.3487, 56.0664) -> (407.4838, 56.0664)
  line L464 (407.4838, 56.0664) -> (407.1333, 61.1464)
  line L465 (407.1333, 61.1464) -> (407.7842, 61.1464)
  line L466 (407.7842, 61.1464) -> (407.9845, 57.6869)
  line L467 (407.9845, 57.6869) -> (408.0437, 56.7401)
  line L468 (408.0437, 56.7401) -> (408.2895, 57.5458)
  line L469 (408.2895, 57.5458) -> (408.904, 59.4303)
  line L470 (408.904, 59.4303) -> (409.382, 59.4303)
  line L471 (409.382, 59.4303) -> (410.0921, 57.4093)
  line L472 (410.0921, 57.4093) -> (410.3288, 56.7401)
  line L473 (410.3288, 56.7401) -> (410.3424, 57.4366)
  line L474 (410.3424, 57.4366) -> (410.5427, 61.1464)
  line L475 (410.5427, 61.1464) -> (411.1618, 61.1464)
  line L476 (415.6819, 56.0664) -> (414.9263, 56.0664)
  line L477 (414.9263, 56.0664) -> (414.5758, 57.1726)
  line L478 (414.5758, 57.1726) -> (412.45, 57.1726)
  line L479 (412.45, 57.1726) -> (412.095, 56.0664)
  line L480 (412.095, 56.0664) -> (411.3803, 56.0664)
  line L481 (411.3803, 56.0664) -> (413.0645, 61.1464)
  line L482 (413.0645, 61.1464) -> (414.0159, 61.1464)
  line L483 (414.0159, 61.1464) -> (415.6819, 56.0664)
  line L484 (414.3755, 57.7916) -> (413.5152, 60.5137)
  line L485 (413.5152, 60.5137) -> (412.6457, 57.7916)
  line L486 (412.6457, 57.7916) -> (414.3755, 57.7916)
  line L487 (323.1449, 47.5006) -> (322.4666, 47.5006)
  line L488 (322.4666, 47.5006) -> (322.4666, 49.9951)
  spline S374 degree 2 poles (322.4666, 49.9951) (322.4666, 50.4457) (322.1298, 50.8918) (321.8157, 50.8918) knots 0 0 0 1 2 2 2
  spline S375 degree 2 poles (321.8157, 50.8918) (321.6791, 50.8918) (321.4424, 50.819) (321.183, 50.6369) (320.8825, 50.3228) (320.6823, 50.0907) knots 0 0 0 1 2 3 4 4 4
  line L489 (320.6823, 50.0907) -> (320.6823, 47.5006)
  line L490 (320.6823, 47.5006) -> (320.004, 47.5006)
  line L491 (320.004, 47.5006) -> (320.004, 52.9949)
  line L492 (320.004, 52.9949) -> (320.6823, 52.9949)
  line L493 (320.6823, 52.9949) -> (320.6823, 51.4062)
  line L494 (320.6823, 51.4062) -> (320.6595, 50.7917)
  spline S376 degree 2 poles (320.6595, 50.7917) (320.8188, 50.9829) (321.1238, 51.2423) (321.4333, 51.4062) (321.752, 51.4745) (321.9249, 51.4745) knots 0 0 0 1 2 3 4 4 4
  spline S377 degree 2 poles (321.9249, 51.4745) (322.5076, 51.4745) (323.1449, 50.7644) (323.1449, 50.0497) knots 0 0 0 1 2 2 2
  line L495 (323.1449, 50.0497) -> (323.1449, 47.5006)
  spline S378 degree 2 poles (327.5284, 47.5552) (327.3008, 47.4961) (326.8092, 47.446) (326.5543, 47.446) knots 0 0 0 1 2 2 2
  spline S379 degree 2 poles (326.5543, 47.446) (325.8214, 47.446) (325.0977, 48.1106) (325.0977, 48.7979) knots 0 0 0 1 2 2 2
  line L496 (325.0977, 48.7979) -> (325.0977, 50.8327)
  line L497 (325.0977, 50.8327) -> (324.0052, 50.8327)
  line L498 (324.0052, 50.8327) -> (324.0052, 51.4017)
  line L499 (324.0052, 51.4017) -> (325.0977, 51.4017)
  line L500 (325.0977, 51.4017) -> (325.0977, 52.4759)
  line L501 (325.0977, 52.4759) -> (325.7759, 52.6489)
  line L502 (325.7759, 52.6489) -> (325.7759, 51.4017)
  line L503 (325.7759, 51.4017) -> (327.5284, 51.4017)
  line L504 (327.5284, 51.4017) -> (327.5284, 50.8327)
  line L505 (327.5284, 50.8327) -> (325.7759, 50.8327)
  line L506 (325.7759, 50.8327) -> (325.7759, 48.8526)
  spline S380 degree 2 poles (325.7759, 48.8526) (325.7759, 48.4338) (326.222, 48.0195) (326.659, 48.0195) knots 0 0 0 1 2 2 2
  spline S381 degree 2 poles (326.659, 48.0195) (326.8456, 48.0195) (327.2872, 48.0787) (327.5284, 48.1379) knots 0 0 0 1 2 2 2
  line L507 (327.5284, 48.1379) -> (327.5284, 47.5552)
  spline S382 degree 2 poles (331.9074, 47.5552) (331.6798, 47.4961) (331.1882, 47.446) (330.9333, 47.446) knots 0 0 0 1 2 2 2
  spline S383 degree 2 poles (330.9333, 47.446) (330.2004, 47.446) (329.4767, 48.1106) (329.4767, 48.7979) knots 0 0 0 1 2 2 2
  line L508 (329.4767, 48.7979) -> (329.4767, 50.8327)
  line L509 (329.4767, 50.8327) -> (328.3842, 50.8327)
  line L510 (328.3842, 50.8327) -> (328.3842, 51.4017)
  line L511 (328.3842, 51.4017) -> (329.4767, 51.4017)
  line L512 (329.4767, 51.4017) -> (329.4767, 52.4759)
  line L513 (329.4767, 52.4759) -> (330.1549, 52.6489)
  line L514 (330.1549, 52.6489) -> (330.1549, 51.4017)
  line L515 (330.1549, 51.4017) -> (331.9074, 51.4017)
  line L516 (331.9074, 51.4017) -> (331.9074, 50.8327)
  line L517 (331.9074, 50.8327) -> (330.1549, 50.8327)
  line L518 (330.1549, 50.8327) -> (330.1549, 48.8526)
  spline S384 degree 2 poles (330.1549, 48.8526) (330.1549, 48.4338) (330.601, 48.0195) (331.038, 48.0195) knots 0 0 0 1 2 2 2
  spline S385 degree 2 poles (331.038, 48.0195) (331.2246, 48.0195) (331.6662, 48.0787) (331.9074, 48.1379) knots 0 0 0 1 2 2 2
  line L519 (331.9074, 48.1379) -> (331.9074, 47.5552)
  spline S386 degree 2 poles (336.473, 49.5217) (336.473, 49.0028) (336.1817, 48.2244) (335.6719, 47.71) (334.9709, 47.4551) (334.5658, 47.4551) knots 0 0 0 1 2 3 4 4 4
  spline S387 degree 2 poles (334.5658, 47.4551) (334.3791, 47.4551) (334.0104, 47.4915) (333.8192, 47.5416) knots 0 0 0 1 2 2 2
  line L520 (333.8192, 47.5416) -> (333.8192, 45.9074)
  line L521 (333.8192, 45.9074) -> (333.141, 45.9074)
  line L522 (333.141, 45.9074) -> (333.141, 51.4017)
  line L523 (333.141, 51.4017) -> (333.7464, 51.4017)
  line L524 (333.7464, 51.4017) -> (333.7874, 50.7507)
  spline S388 degree 2 poles (333.7874, 50.7507) (334.0787, 51.1513) (334.7387, 51.4745) (335.1211, 51.4745) knots 0 0 0 1 2 2 2
  spline S389 degree 2 poles (335.1211, 51.4745) (335.458, 51.4745) (335.9587, 51.1968) (336.3046, 50.687) (336.473, 49.9678) (336.473, 49.5217) knots 0 0 0 1 2 3 4 4 4
  spline S390 degree 2 poles (335.7811, 49.4898) (335.7811, 49.7994) (335.6901, 50.3092) (335.4989, 50.6779) (335.1939, 50.8827) (334.9846, 50.8827) knots 0 0 0 1 2 3 4 4 4
  spline S391 degree 2 poles (334.9846, 50.8827) (334.8571, 50.8827) (334.5931, 50.8008) (334.3109, 50.6096) (333.9968, 50.2955) (333.8192, 50.0634) knots 0 0 0 1 2 3 4 4 4
  line L525 (333.8192, 50.0634) -> (333.8192, 48.1698)
  spline S392 degree 2 poles (333.8192, 48.1698) (334.0059, 48.0924) (334.4156, 48.0013) (334.6158, 48.0013) knots 0 0 0 1 2 2 2
  spline S393 degree 2 poles (334.6158, 48.0013) (335.1621, 48.0013) (335.7811, 48.7433) (335.7811, 49.4898) knots 0 0 0 1 2 2 2
  spline S394 degree 2 poles (340.6062, 48.5658) (340.6062, 48.3609) (340.4651, 48.0332) (340.2239, 47.7828) (339.9052, 47.6053) (339.5456, 47.487) (339.1633, 47.4323) (338.9812, 47.4323) knots 0 0 0 1 2 3 4 5 6 6 6
  spline S395 degree 2 poles (338.9812, 47.4323) (338.5852, 47.4323) (337.9206, 47.5052) (337.6019, 47.5826) knots 0 0 0 1 2 2 2
  line L526 (337.6019, 47.5826) -> (337.6019, 48.2062)
  spline S396 degree 2 poles (337.6019, 48.2062) (337.9433, 48.106) (338.6216, 48.0059) (338.9539, 48.0059) knots 0 0 0 1 2 2 2
  spline S397 degree 2 poles (338.9539, 48.0059) (339.4409, 48.0059) (339.9052, 48.2699) (339.9052, 48.5112) knots 0 0 0 1 2 2 2
  spline S398 degree 2 poles (339.9052, 48.5112) (339.9052, 48.6159) (339.8324, 48.7843) (339.6367, 48.9345) (339.2315, 49.0984) (338.8765, 49.2031) knots 0 0 0 1 2 3 4 4 4
  spline S399 degree 2 poles (338.8765, 49.2031) (338.6125, 49.2804) (338.1664, 49.4807) (337.8386, 49.7538) (337.652, 50.118) (337.652, 50.3684) knots 0 0 0 1 2 3 4 4 4
  spline S400 degree 2 poles (337.652, 50.3684) (337.652, 50.5322) (337.8022, 50.9192) (338.1709, 51.2514) (338.79, 51.4745) (339.2589, 51.4745) knots 0 0 0 1 2 3 4 4 4
  spline S401 degree 2 poles (339.2589, 51.4745) (339.4865, 51.4745) (340.0463, 51.4244) (340.3513, 51.3607) knots 0 0 0 1 2 2 2
  line L527 (340.3513, 51.3607) -> (340.3513, 50.7598)
  spline S402 degree 2 poles (340.3513, 50.7598) (340.0327, 50.8372) (339.4591, 50.91) (339.2498, 50.91) knots 0 0 0 1 2 2 2
  spline S403 degree 2 poles (339.2498, 50.91) (338.9994, 50.91) (338.6534, 50.8327) (338.4395, 50.6961) (338.3439, 50.514) (338.3439, 50.4093) knots 0 0 0 1 2 3 4 4 4
  spline S404 degree 2 poles (338.3439, 50.4093) (338.3439, 50.3046) (338.4258, 50.1317) (338.6489, 49.9723) (339.0449, 49.813) (339.3635, 49.722) knots 0 0 0 1 2 3 4 4 4
  spline S405 degree 2 poles (339.3635, 49.722) (339.7095, 49.6218) (340.1829, 49.3988) (340.4788, 49.1257) (340.6062, 48.7843) (340.6062, 48.5658) knots 0 0 0 1 2 3 4 4 4
  spline S406 degree 2 poles (343.4649, 51.4745) (343.5832, 51.4745) (343.8017, 51.3789) (343.9656, 51.215) (344.0612, 50.9965) (344.0612, 50.8782) knots 0 0 0 1 2 3 4 4 4
  spline S407 degree 2 poles (344.0612, 50.8782) (344.0612, 50.7507) (343.9656, 50.5368) (343.8017, 50.3729) (343.5832, 50.2819) (343.4649, 50.2819) knots 0 0 0 1 2 3 4 4 4
  spline S408 degree 2 poles (343.4649, 50.2819) (343.3374, 50.2819) (343.1235, 50.3729) (342.9596, 50.5368) (342.8686, 50.7507) (342.8686, 50.8782) knots 0 0 0 1 2 3 4 4 4
  spline S409 degree 2 poles (342.8686, 50.8782) (342.8686, 50.9965) (342.9596, 51.215) (343.1235, 51.3789) (343.3374, 51.4745) (343.4649, 51.4745) knots 0 0 0 1 2 3 4 4 4
  spline S410 degree 2 poles (343.4649, 48.625) (343.5832, 48.625) (343.8017, 48.5294) (343.9656, 48.3655) (344.0612, 48.147) (344.0612, 48.0287) knots 0 0 0 1 2 3 4 4 4
  spline S411 degree 2 poles (344.0612, 48.0287) (344.0612, 47.9012) (343.9656, 47.6873) (343.8017, 47.5234) (343.5832, 47.4323) (343.4649, 47.4323) knots 0 0 0 1 2 3 4 4 4
  spline S412 degree 2 poles (343.4649, 47.4323) (343.3374, 47.4323) (343.1235, 47.5234) (342.9596, 47.6873) (342.8686, 47.9012) (342.8686, 48.0287) knots 0 0 0 1 2 3 4 4 4
  spline S413 degree 2 poles (342.8686, 48.0287) (342.8686, 48.147) (342.9596, 48.3655) (343.1235, 48.5294) (343.3374, 48.625) (343.4649, 48.625) knots 0 0 0 1 2 3 4 4 4
  line L528 (349.4143, 52.9949) -> (346.7468, 46.6631)
  line L529 (346.7468, 46.6631) -> (346.1005, 46.6631)
  line L530 (346.1005, 46.6631) -> (348.7679, 52.9949)
  line L531 (348.7679, 52.9949) -> (349.4143, 52.9949)
  line L532 (353.7933, 52.9949) -> (351.1258, 46.6631)
  line L533 (351.1258, 46.6631) -> (350.4795, 46.6631)
  line L534 (350.4795, 46.6631) -> (353.1469, 52.9949)
  line L535 (353.1469, 52.9949) -> (353.7933, 52.9949)
  spline S414 degree 2 poles (357.8446, 50.8509) (357.9538, 50.7143) (358.0722, 50.3547) (358.0722, 50.1453) knots 0 0 0 1 2 2 2
  spline S415 degree 2 poles (358.0722, 50.1453) (358.0722, 49.8403) (357.8491, 49.3396) (357.4485, 48.9846) (356.8841, 48.7843) (356.5472, 48.7843) knots 0 0 0 1 2 3 4 4 4
  spline S416 degree 2 poles (356.5472, 48.7843) (356.3014, 48.7843) (355.8736, 48.889) (355.7506, 48.9664) knots 0 0 0 1 2 2 2
  spline S417 degree 2 poles (355.7506, 48.9664) (355.6733, 48.8571) (355.5731, 48.6659) (355.5731, 48.543) knots 0 0 0 1 2 2 2
  spline S418 degree 2 poles (355.5731, 48.543) (355.5731, 48.3974) (355.8553, 48.2016) (356.092, 48.1925) knots 0 0 0 1 2 2 2
  line L536 (356.092, 48.1925) -> (357.1162, 48.1561)
  spline S419 degree 2 poles (357.1162, 48.1561) (357.4076, 48.147) (357.9037, 48.015) (358.2542, 47.7646) (358.4545, 47.4005) (358.4545, 47.1592) knots 0 0 0 1 2 3 4 4 4
  spline S420 degree 2 poles (358.4545, 47.1592) (358.4545, 46.8998) (358.2269, 46.4309) (357.7581, 46.0759) (357.0343, 45.8665) (356.5381, 45.8665) knots 0 0 0 1 2 3 4 4 4
  spline S421 degree 2 poles (356.5381, 45.8665) (356.0647, 45.8665) (355.4001, 46.0167) (354.9723, 46.2852) (354.7765, 46.654) (354.7765, 46.877) knots 0 0 0 1 2 3 4 4 4
  spline S422 degree 2 poles (354.7765, 46.877) (354.7765, 47.1638) (355.0405, 47.5917) (355.3182, 47.7874) knots 0 0 0 1 2 2 2
  spline S423 degree 2 poles (355.3182, 47.7874) (355.2135, 47.8329) (355.0679, 47.974) (354.9723, 48.1425) (354.9267, 48.3291) (354.9267, 48.4201) knots 0 0 0 1 2 3 4 4 4
  spline S424 degree 2 poles (354.9267, 48.4201) (354.9267, 48.6705) (355.1634, 49.0893) (355.3273, 49.2759) knots 0 0 0 1 2 2 2
  spline S425 degree 2 poles (355.3273, 49.2759) (355.2545, 49.3669) (355.1407, 49.5399) (355.0587, 49.7356) (355.0178, 49.9678) (355.0178, 50.1135) knots 0 0 0 1 2 3 4 4 4
  spline S426 degree 2 poles (355.0178, 50.1135) (355.0178, 50.4184) (355.2408, 50.9192) (355.6414, 51.2742) (356.2013, 51.4745) (356.5427, 51.4745) knots 0 0 0 1 2 3 4 4 4